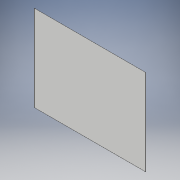
# Autodesk Inventor part: paper
Saved by Autodesk Inventor 2019 (Build 230136000, 136)
## iProperties
Created: 2018-12-01
Part Number: paper
Material: Generic
Document SubType Name: Modeling
Designer: caleb
Density: 1 g/cm^3
Appearance: Default
Author: caleb
Autodesk Inventor part; units mm, degrees
ref_plane "YZ Plane" through (0, 0, 0) normal (1, 0, 0) x (0, 1, 0)
ref_plane "XZ Plane" through (0, 0, 0) normal (0, 1, 0) x (-1, 0, 0)
ref_plane "XY Plane" through (0, 0, 0) normal (0, 0, 1) x (1, 0, 0)
sketch "Sketch1" plane through (0, 0, 0) normal (0, 0, 1) x (1, 0, 0)
  line L0 (-139.7, -107.95) -> (139.7, -107.95)
  line L1 (139.7, -107.95) -> (139.7, 107.95)
  line L2 (139.7, 107.95) -> (-139.7, 107.95)
  line L3 (-139.7, 107.95) -> (-139.7, -107.95)
  line L4 (-139.7, -107.95) -> (139.7, 107.95) construction
  line L5 (139.7, -107.95) -> (-139.7, 107.95) construction
  point P0 (0, 0)
  dimension "d0" = 279.4
  dimension "d1" = 215.9
  constraints: 12 end point, 2 midpoint, 2 parallel, 1 horizontal, 1 perpendicular
  measures "d0" distance of L0.start L0.end
  measures "d1" distance of L2.end L0.start
extrude "Extrusion1" add sketch "Sketch1" along normal blind 0.2
body "Solid1"
